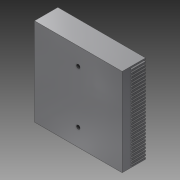
# Autodesk Inventor part: heatsink
Saved by Autodesk Inventor 2018.3 (Build 223284000, 284)
## iProperties
Created: 2019-01-30
Part Number: heatsink
Material: Aluminum 6061
Document SubType Name: Modeling
Designer: callum.snowden
Density: 2.7 g/cm^3
Appearance: Aluminum - Dark
Author: callum.snowden
Autodesk Inventor part; units mm, degrees
ref_plane "YZ Plane" through (0, 0, 0) normal (1, 0, 0) x (0, 1, 0)
ref_plane "XZ Plane" through (0, 0, 0) normal (0, 1, 0) x (-1, 0, 0)
ref_plane "XY Plane" through (0, 0, 0) normal (0, 0, 1) x (1, 0, 0)
sketch "Sketch1" plane through (0, 0, 0) normal (0, 1, 0) x (-1, 0, 0)
  line L0 (0, -72) -> (0, 12) construction
  line L1 (-12, 0) -> (72, 0) construction
  line L2 (0, 0) -> (60, 0)
  line L3 (60, 0) -> (60, -60)
  line L4 (60, -60) -> (0, -60)
  line L5 (0, -60) -> (0, 0)
  dimension "d0" = 60
  dimension "d1" = 60
  constraints: 8 end point, 2 parallel, 1 horizontal, 1 perpendicular
  measures "d0" distance of L3.end L4.end
  measures "d1" distance of L2.end L3.end
extrude "Extrusion1" add sketch "Sketch1" along normal blind 6
sketch "Sketch2" plane through (0, 6, 0) normal (0, 1, 0) x (1, 0, 0)
  line L0 (-60, 0) -> (0, 0) construction
  line L1 (0, 0) -> (0, 60) construction
  line L2 (0, 60) -> (-60, 60) construction
  line L3 (-60, 60) -> (-60, 0) construction
  line L4 (0, 0) -> (0, 60) construction
  line L5 (-60, 0) -> (0, 0)
  line L6 (0, 0) -> (0, 1)
  line L7 (0, 1) -> (-60, 1)
  line L8 (-60, 1) -> (-60, 0)
  line L9 (-60, 2.107) -> (0, 2.107)
  line L10 (0, 2.107) -> (0, 3.107)
  line L11 (0, 3.107) -> (-60, 3.107)
  line L12 (-60, 3.107) -> (-60, 2.107)
  line L13 (-60, 4.214) -> (0, 4.214)
  line L14 (0, 4.214) -> (0, 5.214)
  line L15 (0, 5.214) -> (-60, 5.214)
  line L16 (-60, 5.214) -> (-60, 4.214)
  line L17 (-60, 6.321) -> (0, 6.321)
  line L18 (0, 6.321) -> (0, 7.321)
  line L19 (0, 7.321) -> (-60, 7.321)
  line L20 (-60, 7.321) -> (-60, 6.321)
  line L21 (-60, 8.428) -> (0, 8.428)
  line L22 (0, 8.428) -> (0, 9.428)
  line L23 (0, 9.428) -> (-60, 9.428)
  line L24 (-60, 9.428) -> (-60, 8.428)
  line L25 (-60, 10.535) -> (0, 10.535)
  line L26 (0, 10.535) -> (0, 11.535)
  line L27 (0, 11.535) -> (-60, 11.535)
  line L28 (-60, 11.535) -> (-60, 10.535)
  line L29 (-60, 12.642) -> (0, 12.642)
  line L30 (0, 12.642) -> (0, 13.642)
  line L31 (0, 13.642) -> (-60, 13.642)
  line L32 (-60, 13.642) -> (-60, 12.642)
  line L33 (-60, 14.749) -> (0, 14.749)
  line L34 (0, 14.749) -> (0, 15.749)
  line L35 (0, 15.749) -> (-60, 15.749)
  line L36 (-60, 15.749) -> (-60, 14.749)
  line L37 (-60, 16.856) -> (0, 16.856)
  line L38 (0, 16.856) -> (0, 17.856)
  line L39 (0, 17.856) -> (-60, 17.856)
  line L40 (-60, 17.856) -> (-60, 16.856)
  line L41 (-60, 18.963) -> (0, 18.963)
  line L42 (0, 18.963) -> (0, 19.963)
  line L43 (0, 19.963) -> (-60, 19.963)
  line L44 (-60, 19.963) -> (-60, 18.963)
  line L45 (-60, 21.07) -> (0, 21.07)
  line L46 (0, 21.07) -> (0, 22.07)
  line L47 (0, 22.07) -> (-60, 22.07)
  line L48 (-60, 22.07) -> (-60, 21.07)
  line L49 (-60, 23.177) -> (0, 23.177)
  line L50 (0, 23.177) -> (0, 24.177)
  line L51 (0, 24.177) -> (-60, 24.177)
  line L52 (-60, 24.177) -> (-60, 23.177)
  line L53 (-60, 25.284) -> (0, 25.284)
  line L54 (0, 25.284) -> (0, 26.284)
  line L55 (0, 26.284) -> (-60, 26.284)
  line L56 (-60, 26.284) -> (-60, 25.284)
  line L57 (-60, 27.391) -> (0, 27.391)
  line L58 (0, 27.391) -> (0, 28.391)
  line L59 (0, 28.391) -> (-60, 28.391)
  line L60 (-60, 28.391) -> (-60, 27.391)
  line L61 (-60, 29.498) -> (0, 29.498)
  line L62 (0, 29.498) -> (0, 30.498)
  line L63 (0, 30.498) -> (-60, 30.498)
  line L64 (-60, 30.498) -> (-60, 29.498)
  line L65 (-60, 31.605) -> (0, 31.605)
  line L66 (0, 31.605) -> (0, 32.605)
  line L67 (0, 32.605) -> (-60, 32.605)
  line L68 (-60, 32.605) -> (-60, 31.605)
  line L69 (-60, 33.712) -> (0, 33.712)
  line L70 (0, 33.712) -> (0, 34.712)
  line L71 (0, 34.712) -> (-60, 34.712)
  line L72 (-60, 34.712) -> (-60, 33.712)
  line L73 (-60, 35.819) -> (0, 35.819)
  line L74 (0, 35.819) -> (0, 36.819)
  line L75 (0, 36.819) -> (-60, 36.819)
  line L76 (-60, 36.819) -> (-60, 35.819)
  line L77 (-60, 37.926) -> (0, 37.926)
  line L78 (0, 37.926) -> (0, 38.926)
  line L79 (0, 38.926) -> (-60, 38.926)
  line L80 (-60, 38.926) -> (-60, 37.926)
  line L81 (-60, 40.033) -> (0, 40.033)
  line L82 (0, 40.033) -> (0, 41.033)
  line L83 (0, 41.033) -> (-60, 41.033)
  line L84 (-60, 41.033) -> (-60, 40.033)
  line L85 (-60, 42.14) -> (0, 42.14)
  line L86 (0, 42.14) -> (0, 43.14)
  line L87 (0, 43.14) -> (-60, 43.14)
  line L88 (-60, 43.14) -> (-60, 42.14)
  line L89 (-60, 44.247) -> (0, 44.247)
  line L90 (0, 44.247) -> (0, 45.247)
  line L91 (0, 45.247) -> (-60, 45.247)
  line L92 (-60, 45.247) -> (-60, 44.247)
  line L93 (-60, 46.354) -> (0, 46.354)
  line L94 (0, 46.354) -> (0, 47.354)
  line L95 (0, 47.354) -> (-60, 47.354)
  line L96 (-60, 47.354) -> (-60, 46.354)
  line L97 (-60, 48.461) -> (0, 48.461)
  line L98 (0, 48.461) -> (0, 49.461)
  line L99 (0, 49.461) -> (-60, 49.461)
  line L100 (-60, 49.461) -> (-60, 48.461)
  line L101 (-60, 50.568) -> (0, 50.568)
  line L102 (0, 50.568) -> (0, 51.568)
  line L103 (0, 51.568) -> (-60, 51.568)
  line L104 (-60, 51.568) -> (-60, 50.568)
  line L105 (-60, 52.675) -> (0, 52.675)
  line L106 (0, 52.675) -> (0, 53.675)
  line L107 (0, 53.675) -> (-60, 53.675)
  line L108 (-60, 53.675) -> (-60, 52.675)
  line L109 (-60, 54.782) -> (0, 54.782)
  line L110 (0, 54.782) -> (0, 55.782)
  line L111 (0, 55.782) -> (-60, 55.782)
  line L112 (-60, 55.782) -> (-60, 54.782)
  line L113 (-60, 56.889) -> (0, 56.889)
  line L114 (0, 56.889) -> (0, 57.889)
  line L115 (0, 57.889) -> (-60, 57.889)
  line L116 (-60, 57.889) -> (-60, 56.889)
  line L117 (-60, 58.996) -> (0, 58.996)
  line L118 (0, 58.996) -> (0, 59.996)
  line L119 (0, 59.996) -> (-60, 59.996)
  line L120 (-60, 59.996) -> (-60, 58.996)
  line L121 (-60, 61.103) -> (0, 61.103)
  line L122 (0, 61.103) -> (0, 62.103)
  line L123 (0, 62.103) -> (-60, 62.103)
  line L124 (-60, 62.103) -> (-60, 61.103)
  line L125 (-60, 63.21) -> (0, 63.21)
  line L126 (0, 63.21) -> (0, 64.21)
  line L127 (0, 64.21) -> (-60, 64.21)
  line L128 (-60, 64.21) -> (-60, 63.21)
  line L129 (-60, 65.317) -> (0, 65.317)
  line L130 (0, 65.317) -> (0, 66.317)
  line L131 (0, 66.317) -> (-60, 66.317)
  line L132 (-60, 66.317) -> (-60, 65.317)
  dimension "d4" = 1
  dimension "d7" = 2.107
  constraints: 256 end point, 2 parallel, 1 horizontal, 1 perpendicular, 1 point on line, 1 vertical, 248 other
  measures "d4" distance of L6.end L5.end
  measures "d7" distance of L6.end L10.end
extrude "Extrusion2" add sketch "Sketch2" along normal blind 10 contours L8 L7 L6 L5 | L12 L11 L10 L9 | L16 L15 L14 L13 | L20 L19 L18 L17 | L24 L23 L22 L21 | L28 L27 L26 L25 | L32 L31 L30 L29 | L36 L35 L34 L33 | L40 L39 L38 L37 | L44 L43 L42 L41 | L48 L47 L46 L45 | L52 L51 L50 L49 | L56 L55 L54 L53 | L60 L59 L58 L57 | L64 L63 L62 L61 | L68 L67 L66 L65 | L72 L71 L70 L69 | L76 L75 L74 L73 | L80 L79 L78 L77 | L84 L83 L82 L81 | L88 L87 L86 L85 | L92 L91 L90 L89 | L96 L95 L94 L93 | L100 L99 L98 L97 | L104 L103 L102 L101 | L108 L107 L106 L105 | L112 L111 L110 L109 | L116 L115 L114 L113 | L120 L119 L118 L117
sketch "Sketch3" plane through (0, 0, 0) normal (0, -1, 0) x (1, 0, 0)
  line L0 (0, 0) -> (-60, 0) construction
  line L1 (-60, 0) -> (-60, -60) construction
  line L2 (-60, -60) -> (0, -60) construction
  line L3 (0, -60) -> (0, 0) construction
  line L4 (-60, -30.498) -> (-60, -29.498) construction
  line L5 (-60, -29.998) -> (0, -30) construction
  line L6 (-60, -60) -> (0, -60) construction
  line L7 (-30, -60) -> (-30, 0) construction
  line L8 (0, 0) -> (-60, 0) construction
  point P0 (-30.0012, -47.999)
  point P1 (-30, -11.999)
  dimension "d17" = 36
  constraints: 4 end point, 4 midpoint, 1 point on line, 1 symmetric about line
  measures "d17" distance of point (-30, -11.999) point (-30.001, -47.999)
hole "Hole1" at (-30.0012, 0, -47.999) at (-30, 0, -11.999) direction (0, 1, 0) diameter 2.459 depth 6 tip angle 118 thread size "M3x0.5" class "6H" standard "ISO Metric profile"
body "Solid1"
